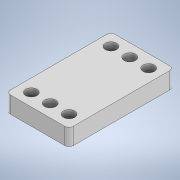
# Autodesk Inventor part: ViseB
Saved by Autodesk Inventor 2022 (Build 260153000, 153)
## iProperties
Created: 2021-11-10
Part Number: ViseB
Material: Genérico
Document SubType Name: Modeling
Designer: JK
Density: 1 g/cm^3
Appearance: Valor por defecto
Author: JK
Autodesk Inventor part; units mm, degrees
ref_plane "YZ Plane" through (0, 0, 0) normal (1, 0, 0) x (0, 1, 0)
ref_plane "XZ Plane" through (0, 0, 0) normal (0, 1, 0) x (-1, 0, 0)
ref_plane "XY Plane" through (0, 0, 0) normal (0, 0, 1) x (1, 0, 0)
sketch "Boceto1" plane through (0, 0, 0) normal (0, 1, 0) x (-1, 0, 0)
  line L0 (-15, 25) -> (15, 25)
  line L1 (15, 25) -> (15, -25)
  line L2 (15, -25) -> (-15, -25)
  line L3 (-15, -25) -> (-15, 25)
  line L4 (-15, 25) -> (15, -25) construction
  line L5 (15, 25) -> (-15, -25) construction
  point P0 (0, 0)
  dimension "d0" = 50
  dimension "d1" = 30
  constraints: 12 end point, 2 midpoint, 2 parallel, 1 horizontal, 1 perpendicular
  measures "d0" distance of L0.end L1.end
  measures "d1" distance of L1.end L2.end
extrude "Extrusión1" add sketch "Boceto1" along normal blind 8
fillet "Empalme1" radius 2 4 edges at (15, 4, 25) (-15, 4, 25) (15, 4, -25) (-15, 4, -25)
sketch "Boceto2" plane through (0, 8, 0) normal (0, 1, 0) x (1, 0, 0)
  circle A0 centre (-9, 19) radius 2.7
  circle A1 centre (9, 19) radius 2.7
  circle A2 centre (9, -19) radius 2.7
  circle A3 centre (-9, -19) radius 2.7
  line L0 (13, 25) -> (-13, 25) projected
  line L1 (-15, 23) -> (-15, -23) projected
  line L2 (15, -23) -> (15, 23) projected
  line L3 (-13, -25) -> (13, -25) projected
  point P0 (0, 0)
  dimension "d5" = 5.4
  dimension "d6" = 6
  dimension "d7" = 6
  dimension "d8" = 6
  dimension "d9" = 6
  constraints: 4 centre point, 3 equal radius, 2 horizontal alignment, 2 vertical alignment
  measures "d5" diameter of A0
  measures "d6" distance from line of L0 A0.centre
  measures "d7" distance from line of L1 A0.centre
  measures "d8" distance from line of L2 A1.centre
  measures "d9" distance from line of L3 A2.centre
extrude "Extrusión2" cut sketch "Boceto2" against normal blind 3
sketch "Boceto3" plane through (0, 0, 0) normal (0, -1, 0) x (1, 0, 0)
  circle A0 centre (0, 19) radius 2.7
  circle A1 centre (0, -19) radius 2.7
  circle A2 centre (-9, -19) radius 2.7 projected
  circle A3 centre (-9, 19) radius 2.7 projected
  point P0 (0, 0)
  dimension "d12" = 5.4
  constraints: 2 centre point, 2 horizontal alignment, 2 vertical alignment, 1 equal radius
  measures "d12" diameter of A1
extrude "Extrusión3" cut sketch "Boceto3" against normal through all contours A0 | A1
sketch "Boceto4" plane through (0, 0, 0) normal (0, -1, 0) x (1, 0, 0)
  circle A0 centre (0, -19) radius 2.7 projected
  circle A1 centre (0, -19) radius 4.05
  line L0 (2.3383, -14.95) -> (4.6765, -19)
  line L1 (4.6765, -19) -> (2.3383, -23.05)
  line L2 (2.3383, -23.05) -> (-2.3383, -23.05)
  line L3 (-2.3383, -23.05) -> (-4.6765, -19)
  line L4 (-4.6765, -19) -> (-2.3383, -14.95)
  line L5 (-2.3383, -14.95) -> (2.3383, -14.95)
  circle A2 centre (0, 19) radius 4.05
  line L6 (-4.6765, 19) -> (-2.3383, 23.05)
  line L7 (-2.3383, 23.05) -> (2.3383, 23.05)
  line L8 (2.3383, 23.05) -> (4.6765, 19)
  line L9 (4.6765, 19) -> (2.3383, 14.95)
  line L10 (2.3383, 14.95) -> (-2.3383, 14.95)
  line L11 (-2.3383, 14.95) -> (-4.6765, 19)
  point P0 (0, 0)
  dimension "d15" = 8.1
  constraints: 24 end point, 4 coincident, 2 centre point, 2 horizontal, 2 tangent, 1 equal radius, 26 other
  measures "d15" diameter of A1
extrude "Extrusión4" cut sketch "Boceto4" against normal blind 4.5 contours A0 | A1 | A1 L0 L1 | A1 L5 L0 | L1 L2 A1 | A1 L4 L5 | L2 L3 A1 | A1 L3 L4 | A2 | A2 L8 L9 | A2 L7 L8 | L9 L10 A2 | A2 L6 L7 | L10 L11 A2 | A2 L11 L6
